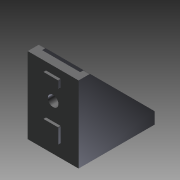
# Autodesk Inventor part: HBLFSN5-4hblfsn5
Saved by Autodesk Inventor 2015 SP1 (Build 190203100, 203)
## iProperties
Category: Hardware
Company: MISUMI
Created: 2015-01-28
Part Number: HBLFSN5-4hblfsn5
Catalog Web Link: http://us.misumi-ec.com/vona2/detail/110300437260/
Description: HBLFSN5, HBLFSNB5, HBLFSNM5, HBLFSNK5, HBLFSSW5, HBLFSSWB5, HBLFSDW5-Thin Reversal Brackets for Slot Width 6 Frames - For 20, 40mm Sections
Vendor: MISUMI
Document SubType Name: Modeling
Designer: psAdmin
Manufacturer: MISUMI
Mass: 6.31246 g
Surface Area: 43.3234 cm^2
Volume: 6.31246 cm^3
Density: 1 g/cm^3
Material: Generic
Appearance: PSOLRGB-192-192-192
PSOL_IDENT_0: {\\10.0.0.236\data_v8\23d-libs\misumi\metric\38_al_extrusions_blackets\5\hblfsn5.prj},246 {VTYP=3D},
PSOL_IDENT_1: {NB=HBLFSN5-4hblfsn5},{LINA=HBLFSN5-4hblfsn5},{NN=HBLFSN5, HBLFSNB5, HBLFSNM5, HBLFSNK5, HBLFSSW5, H
PSOL_IDENT_2: BLFSSWB5, HBLFSDW5},{DATE=19.11.2014 02:27:22},{GEOMDATE=28.01.2010 06:29:00},{VERSION=},{LINEID=290
PSOL_IDENT_3: },{LINESUBID=-1},{WBVAR=ALT1,ALT2}  {NB=HBLFSN5-4hblfsn5},{LINA=HBLFSN5-4hblfsn5},{KT=1},{PN=HBLFSN5
PSOL_IDENT_4: -4},{TP=HBLFSN5-4},{NOH=1},{NOHV=2},{MAT=JIS-ADC12},{ST=-},{TYPE=HBLFSN5-4},{FEAT=Thin Reversal Brac
PSOL_IDENT_5: ket},{ALT1=},{ALT2=},{MASS=15},{AB=CBM4-10},{NOB=2},{AN=HNTT5-4},{NON=2},{AL=1176},{W=20},{H=30},{DP=
PSOL_IDENT_6: 30},{T=4.5},{HDIS=8},{DPOS=12},{HH1=18},{BOLTX=0.0},{HV1=10},{BOLTY=0.0},{DIA=4.2},{ALT1OPT='','w/o
PSOL_IDENT_7: C (Mounting Holes for Cover)','-C','with C (Mounting Holes for Cover)'},{ALT2OPT= '' , 'w/o Set Appl
PSOL_IDENT_8: icable Bolt & Nut' , '-SET' , 'with SET (Set Applicable Bolt & Nut)' , '-SST' , 'with SST (Stainless
PSOL_IDENT_9: Steel Set Applicable Bolt & Nut)' , '-SEP' , 'with SEP (Post Assembly Spring Nuts Set Applicable Bo
PSOL_IDENT_10: lt & Nut)' , '-SSP' , 'with SSP (Post Assembly Spring Nuts, Stainless Steel Set Applicable Bolt & Nu
PSOL_IDENT_11: t)' },{R=1},{R1=0.3},{APOSV=0},{VER=1},{PR=1},{TT=1.0},{T1=1}
SUPPLIER: MISUMI
ARTICLENO: HBLFSN5-4hblfsn5
BOMINFO: HBLFSN5-4hblfsn5
CREATOR: CADENAS GmbH
Title: Extrusion Brace
Author: Misumi
Autodesk Inventor part; units mm, degrees
ref_plane "YZ Plane" through (0, 0, 0) normal (1, 0, 0) x (0, 1, 0)
ref_plane "XZ Plane" through (0, 0, 0) normal (0, 1, 0) x (-1, 0, 0)
ref_plane "XY Plane" through (0, 0, 0) normal (0, 0, 1) x (1, 0, 0)
sketch "Sketch_15" plane through (0, 0, 0) normal (1, 0, 0) x (0, 1, 0)
  line L0 (0, 30) -> (0, 0)
  line L1 (0, 0) -> (30, 0)
  line L2 (30, 0) -> (30, 4.0858)
  arc A0 (30, 4.0858) -> (29.7071, 4.7929) centre (29, 4.0858) ccw
  line L3 (29.7071, 4.7929) -> (4.7929, 29.7071)
  arc A1 (4.7929, 29.7071) -> (4.0858, 30) centre (4.0858, 29) ccw
  line L4 (4.0858, 30) -> (0, 30)
  constraints: 10 end point, 4 point on circle, 2 centre point
extrude "Extrusion1" add sketch "Sketch_15" along normal mid plane 20
sketch "Sketch_16" plane through (0, 0, 0) normal (1, 0, 0) x (0, 1, 0)
  line L0 (2.9278, 34.5) -> (4.5, 4.5)
  line L1 (4.5, 4.5) -> (34.5, 4.5)
  line L2 (34.5, 4.5) -> (34.5, 34.5)
  line L3 (34.5, 34.5) -> (2.9278, 34.5)
  constraints: 8 end point
extrude "Extrusion2" cut sketch "Sketch_16" along normal mid plane 15
sketch "Sketch_17" plane through (0, 4.5, 0) normal (0, 1, 0) x (1, 0, 0)
  line L0 (-5.4209, -10.5) -> (-4.4687, -18.5299)
  arc A0 (-4.4687, -18.5299) -> (4.4687, -18.5299) centre (0, -18) ccw
  line L1 (4.4687, -18.5299) -> (5.4209, -10.5)
  line L2 (5.4209, -10.5) -> (-5.4209, -10.5)
  constraints: 6 end point, 2 point on circle, 1 centre point
extrude "Extrusion3" add sketch "Sketch_17" against normal blind 2.25
sketch "Sketch_2" plane through (0, 0, 0) normal (0, 0, 1) x (1, 0, 0)
  circle A0 centre (0, 18) radius 2.1
  constraints: 1 centre point
extrude "Extrusion4" cut sketch "Sketch_2" along normal blind 4.5
sketch "Sketch_9" plane through (0, 0, 0) normal (0, 0, 1) x (1, 0, 0)
  circle A0 centre (0, 10) radius 2.1
  constraints: 1 centre point
extrude "Extrusion5" cut sketch "Sketch_9" along normal blind 4.5
sketch "Sketch_3" plane through (0, 0, 0) normal (0, 1, 0) x (-1, 0, 0)
  circle A0 centre (0, 18) radius 2.1
  constraints: 1 centre point
extrude "Extrusion6" cut sketch "Sketch_3" along normal blind 4.5
sketch "Sketch_1" plane through (0, 0, 0) normal (0, 1, 0) x (-1, 0, 0)
  line L0 (10, 0) -> (10, 30)
  line L1 (10, 30) -> (-10, 30)
  line L2 (-10, 30) -> (-10, 0)
  line L3 (-10, 0) -> (10, 0)
  constraints: 8 end point
extrude "Extrusion7" add sketch "Sketch_1" against normal blind 1
sketch "Sketch_4" plane through (0, 0, 0) normal (0, 1, 0) x (-1, 0, 0)
  line L0 (10, 0) -> (10, 30)
  line L1 (10, 30) -> (-10, 30)
  line L2 (-10, 30) -> (-10, 0)
  line L3 (-10, 0) -> (10, 0)
  arc A0 (3, 10.7) -> (2.7, 11) centre (2.7, 10.7) ccw
  line L4 (2.7, 11) -> (-2.7, 11)
  arc A1 (-2.7, 11) -> (-3, 10.7) centre (-2.7, 10.7) ccw
  line L5 (-3, 10.7) -> (-3, 5.3)
  arc A2 (-3, 5.3) -> (-2.7, 5) centre (-2.7, 5.3) ccw
  line L6 (-2.7, 5) -> (2.7, 5)
  arc A3 (2.7, 5) -> (3, 5.3) centre (2.7, 5.3) ccw
  line L7 (3, 5.3) -> (3, 10.7)
  arc A4 (3, 26.7) -> (2.7, 27) centre (2.7, 26.7) ccw
  line L8 (2.7, 27) -> (-2.7, 27)
  arc A5 (-2.7, 27) -> (-3, 26.7) centre (-2.7, 26.7) ccw
  line L9 (-3, 26.7) -> (-3, 24.3)
  arc A6 (-3, 24.3) -> (-2.7, 24) centre (-2.7, 24.3) ccw
  line L10 (-2.7, 24) -> (2.7, 24)
  arc A7 (2.7, 24) -> (3, 24.3) centre (2.7, 24.3) ccw
  line L11 (3, 24.3) -> (3, 26.7)
  constraints: 24 end point, 16 point on circle, 8 centre point
extrude "Extrusion8" cut sketch "Sketch_4" against normal blind 1
sketch "Sketch_10" plane through (0, 0, 0) normal (0, 0, 1) x (1, 0, 0)
  line L0 (-10, 0) -> (10, 0)
  line L1 (10, 0) -> (10, 30)
  line L2 (10, 30) -> (-10, 30)
  line L3 (-10, 30) -> (-10, 0)
  constraints: 8 end point
extrude "Extrusion9" add sketch "Sketch_10" against normal blind 1
sketch "Sketch_11" plane through (0, 0, 0) normal (0, 0, 1) x (1, 0, 0)
  line L0 (-10, 0) -> (10, 0)
  line L1 (10, 0) -> (10, 30)
  line L2 (10, 30) -> (-10, 30)
  line L3 (-10, 30) -> (-10, 0)
  line L4 (0.5, 7) -> (2, 7)
  arc A0 (2, 7) -> (3, 8) centre (2, 8) ccw
  line L5 (3, 8) -> (3, 9.5)
  line L6 (3, 9.5) -> (2.0396, 9.5)
  arc A1 (0.5, 7.9604) -> (2.0396, 9.5) centre (0, 10) ccw
  line L7 (0.5, 7.9604) -> (0.5, 7)
  line L8 (0.5, 13) -> (0.5, 12.0396)
  arc A2 (2.0396, 10.5) -> (0.5, 12.0396) centre (0, 10) ccw
  line L9 (2.0396, 10.5) -> (3, 10.5)
  line L10 (3, 10.5) -> (3, 12)
  arc A3 (3, 12) -> (2, 13) centre (2, 12) ccw
  line L11 (2, 13) -> (0.5, 13)
  line L12 (-3, 9.5) -> (-3, 8)
  arc A4 (-3, 8) -> (-2, 7) centre (-2, 8) ccw
  line L13 (-2, 7) -> (-0.5, 7)
  line L14 (-0.5, 7) -> (-0.5, 7.9604)
  arc A5 (-2.0396, 9.5) -> (-0.5, 7.9604) centre (0, 10) ccw
  line L15 (-2.0396, 9.5) -> (-3, 9.5)
  line L16 (-3, 10.5) -> (-2.0396, 10.5)
  arc A6 (-0.5, 12.0396) -> (-2.0396, 10.5) centre (0, 10) ccw
  line L17 (-0.5, 12.0396) -> (-0.5, 13)
  line L18 (-0.5, 13) -> (-2, 13)
  arc A7 (-2, 13) -> (-3, 12) centre (-2, 12) ccw
  line L19 (-3, 12) -> (-3, 10.5)
  constraints: 40 end point, 16 point on circle, 8 centre point
extrude "Extrusion10" cut sketch "Sketch_11" against normal blind 1
body "Solid1"
